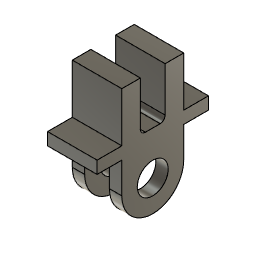
Exercise_3 v1 (Autodesk Fusion 360 design; units mm, degrees)
Autodesk Fusion 360 part; units mm, degrees
sketch "Sketch1" plane through (0, 0, 0) normal (0, 0, 1) x (1, 0, 0)
  line L0 (-10, 22.5) -> (10, 22.5)
  line L1 (10, 22.5) -> (10, -22.5)
  line L2 (10, -22.5) -> (-10, -22.5)
  line L3 (-10, -22.5) -> (-10, 22.5)
  line L4 (10, 12.5) -> (5, 12.5)
  line L5 (5, 12.5) -> (5, -12.5)
  line L6 (5, -12.5) -> (10, -12.5)
  line L7 (10, -12.5) -> (10, 12.5)
  line L8 (0, 22.5) -> (0, -22.5)
  line L9 (-10, 22.5) -> (-10, -22.5)
  line L10 (-10, -12.5) -> (-10, 12.5)
  line L11 (-5, -12.5) -> (-10, -12.5)
  line L12 (-5, 12.5) -> (-5, -12.5)
  line L13 (-10, 0) -> (10, 0)
  line L14 (-10, 12.5) -> (10, 12.5)
  line L15 (10, 12.5) -> (10, 5)
  line L16 (10, 5) -> (-10, 5)
  line L17 (-10, 5) -> (-10, 12.5)
  line L18 (10, -5) -> (-10, -5)
  line L19 (-10, -12.5) -> (10, -12.5)
  dimension "d1" = 20
  dimension "d2" = 45
  dimension "d3" = 22.5
  dimension "d4" = 10
  dimension "d5" = 5
  dimension "d6" = 25
  dimension "d7" = 12.5
  dimension "d8" = 7.5
  dimension "d9" = 10
  constraint horizontal L0
  constraint vertical L1
  constraint horizontal L2
  constraint vertical L3
  constraint horizontal L4
  constraint vertical L5
  constraint horizontal L6
  constraint vertical L7
  constraint coincident L1 L4.start
  constraint midpoint L0 L8.start
  constraint midpoint L2 L8.end
  constraint symmetric L0.end L8 L0.start
  constraint symmetric L1.end L8 L2.end
  constraint symmetric L4.start L8 L10.end
  constraint symmetric L4.end L8 L12.start
  constraint symmetric L5.end L8 L11.start
  constraint symmetric L6.end L8 L10.start
  constraint midpoint L10 L13.start
  constraint midpoint L1 L13.end
  constraint horizontal L14
  constraint vertical L15
  constraint horizontal L16
  constraint vertical L17
  constraint coincident L1 L15.end
  constraint coincident L9 L10.end
  constraint symmetric L13 L10.end L10.start
  constraint symmetric L13 L4.start L6.end
  constraint symmetric L13 L15.end L18.start
  constraint symmetric L13 L16.end L18.end
  measures "d1" distance of L0.start L0.end
  measures "d2" distance of L0.end L1.end
  measures "d3" distance of origin L2
  measures "d4" distance of origin L1
  measures "d5" distance of L4.start L4.end
  measures "d6" distance of L4.end L5.end
  measures "d7" distance of origin L4
  measures "d8" distance of L4.start L15.end
  measures "d9" distance of L0.end L14
extrude "Extrude1" add sketch "Sketch1" along normal blind 25 contours L3 L9 L10 L12 L14 L16 L17 | L5 L8 L14 L16 | L8 L12 L14 L16 | L1 L4 L5 L7 L14 L15 L16 | L3 L9 L10 L11 L12 L18 L19 | L5 L8 L18 L19 | L8 L12 L18 L19 | L1 L5 L6 L7 L18 L19 makes body 1 at (-3.3333, 12.5, 8.3333) makes body 2 at (3.3333, -5, 8.3333)
extrude "Extrude2" add sketch "Sketch1" against normal blind 25 contours L3 L9 L10 L12 L14 L16 L17 | L3 L9 L10 L12 L13 L16 | L1 L4 L5 L7 L14 L15 L16 | L3 L9 L10 L12 L13 L18 | L1 L5 L7 L13 L16 | L3 L9 L10 L11 L12 L18 L19 | L1 L5 L7 L13 L18 | L1 L5 L6 L7 L18 L19 bodies 1 2
extrude "Extrude3" add sketch "Sketch1" along normal blind 5 contours L0 L3 L8 L9 L14 | L0 L1 L4 L8 L14 | L3 L9 L10 L12 L13 L16 | L5 L8 L13 L16 | L8 L12 L13 L16 | L3 L9 L10 L12 L13 L18 | L1 L5 L7 L13 L16 | L5 L8 L13 L18 | L8 L12 L13 L18 | L1 L5 L7 L13 L18 | L2 L3 L8 L9 L11 L19 | L1 L2 L6 L8 L19 bodies 1
fillet "Fillet1" radius 12.5 4 edges at (7.5, -12.5, -25) (-7.5, -12.5, -25) (-7.5, 12.5, -25) (7.5, 12.5, -25) on bodies 1
fillet "Fillet2" radius 2 2 edges at (0, -5, 5) (0, 5, 5) on bodies 1
sketch "Sketch2" plane through (10, 0, 0) normal (1, 0, 0) x (0, 1, 0)
  arc A0 (-12.5, -12.5) -> (12.5, -12.5) centre (0, -12.5) ccw
  line L0 (12.5, -12.5) -> (12.5, 0)
  line L1 (12.5, 0) -> (22.5, 0)
  line L2 (22.5, 0) -> (22.5, 5)
  line L3 (22.5, 5) -> (12.5, 5)
  line L4 (12.5, 5) -> (12.5, 25)
  line L5 (12.5, 25) -> (5, 25)
  line L6 (5, 25) -> (5, 7)
  arc A1 (3, 5) -> (5, 7) centre (3, 7) ccw
  line L7 (3, 5) -> (-3, 5)
  arc A2 (-5, 7) -> (-3, 5) centre (-3, 7) ccw
  line L8 (-5, 7) -> (-5, 25)
  line L9 (-5, 25) -> (-12.5, 25)
  line L10 (-12.5, 25) -> (-12.5, 5)
  line L11 (-12.5, 5) -> (-22.5, 5)
  line L12 (-22.5, 5) -> (-22.5, 0)
  line L13 (-22.5, 0) -> (-12.5, 0)
  line L14 (-12.5, 0) -> (-12.5, -12.5)
  circle A3 centre (0, -12.5) radius 6.25
  dimension "d20" = 12.5
  dimension "d21" = 12.5
  measures "d20" diameter of A3
  measures "d21" distance of A0.centre origin
extrude "Extrude4" cut sketch "Sketch2" against normal up to surface (20 mm away) contours A3 bodies 1
equation "d3 = ( 45 / 2 ) * 1 mm"
equation "d7 = ( 25 / 2 ) * 1 mm"
equation "d8 = ( 15 / 2 ) * 1 mm"
